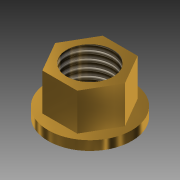
# Autodesk Inventor part: 刮肉轮固定螺丝
Saved by Autodesk Inventor 2015 (Build 190159000, 159)
## iProperties
Created: 2017-05-22
Part Number: 刮肉轮固定螺丝
Material: 常规
Document SubType Name: Modeling
Designer: Administrator
Density: 1 g/cm^3
Appearance: 黄铜 - 抛光
Author: Administrator
Autodesk Inventor part; units mm, degrees
ref_plane "YZ Plane" through (0, 0, 0) normal (1, 0, 0) x (0, 1, 0)
ref_plane "XZ Plane" through (0, 0, 0) normal (0, 1, 0) x (-1, 0, 0)
ref_plane "XY Plane" through (0, 0, 0) normal (0, 0, 1) x (1, 0, 0)
sketch "草图1" plane through (0, 0, 0) normal (0, 0, 1) x (1, 0, 0)
  circle A0 centre (0, 0) radius 4.5
  dimension "d0" = 9
  constraints: 1 centre point, 1 coincident
  measures "d0" diameter of A0
extrude "拉伸1" add sketch "草图1" along normal blind 1
sketch "草图2" plane through (0, 0, 1) normal (0, 0, 1) x (1, 0, 0)
  line L0 (1.8764, -3.25) -> (-1.8764, -3.25)
  line L1 (-1.8764, -3.25) -> (-3.7528, 0)
  line L2 (-3.7528, 0) -> (-1.8764, 3.25)
  line L3 (-1.8764, 3.25) -> (1.8764, 3.25)
  line L4 (1.8764, 3.25) -> (3.7528, 0)
  line L5 (3.7528, 0) -> (1.8764, -3.25)
  line L6 (0, 0) -> (0, 3.25)
  dimension "d3" = 6.5
  constraints: 14 end point, 1 coincident, 1 midpoint, 1 vertical, 13 other
  measures "d3" distance between parallel lines of L0 L3
extrude "拉伸2" add sketch "草图2" along normal blind 4
sketch "草图3" plane through (0, 0, 5) normal (0, 0, 1) x (1, 0, 0)
  circle A0 centre (0, 0) radius 2.5
  dimension "d6" = 5
  constraints: 1 centre point, 1 coincident
  measures "d6" diameter of A0
extrude "拉伸3" cut sketch "草图3" against normal through all
thread "螺纹1" size "M5x0.8" class "6H" standard "ANSI Metric M Profile" full length
